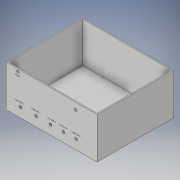
# Autodesk Inventor part: SeniorProjects
Saved by Autodesk Inventor 2019 (Build 230136000, 136)
## iProperties
Created: 2019-02-05
Part Number: SeniorProjects
Material: Generic
Document SubType Name: Modeling
Designer: Austin
Density: 1 g/cm^3
Appearance: Default
Author: Austin
Autodesk Inventor part; units mm, degrees
ref_plane "YZ Plane" through (0, 0, 0) normal (1, 0, 0) x (0, 1, 0)
ref_plane "XZ Plane" through (0, 0, 0) normal (0, 1, 0) x (-1, 0, 0)
ref_plane "XY Plane" through (0, 0, 0) normal (0, 0, 1) x (1, 0, 0)
sketch "Sketch1" plane through (0, 0, 0) normal (0, 1, 0) x (-1, 0, 0)
  line L0 (0, 0) -> (-203.2, 0)
  line L1 (-203.2, 0) -> (-203.2, 171.45)
  line L2 (-203.2, 171.45) -> (0, 171.45)
  line L3 (0, 171.45) -> (0, 0)
  dimension "d47" = 203.2
  dimension "d48" = 171.45
  constraints: 8 end point, 2 parallel, 1 horizontal, 1 perpendicular
  measures "d47" distance of L1.end L2.end
  measures "d48" distance of L0.end L1.end
extrude "Extrusion1" add sketch "Sketch1" along normal blind 2.54
sketch "Sketch2" plane through (0, 2.54, 0) normal (0, 1, 0) x (1, 0, 0)
  point P0 (0, 0)
sketch "Sketch3" plane through (203.2, 0, 171.45) normal (1, 0, 0) x (0, 0, -1)
  line L0 (171.45, 2.54) -> (0, 2.54) projected
  line L1 (0, 2.54) -> (171.4319, 2.54)
  line L2 (171.4319, 2.54) -> (171.4319, 92.0353)
  line L3 (171.4319, 92.0353) -> (0, 92.0353)
  line L4 (0, 92.0353) -> (0, 2.54)
  point P0 (171.45, 0)
  constraints: 8 end point, 2 parallel, 1 horizontal, 1 perpendicular
extrude "Extrusion2" add sketch "Sketch3" against normal blind 2.54
sketch "Sketch4" plane through (0, 0, 171.45) normal (0, 0, 1) x (1, 0, 0)
  line L0 (200.66, 2.54) -> (0, 2.54) projected
  line L1 (200.66, 92.0353) -> (200.66, 2.54) projected
  line L2 (0, 2.54) -> (200.66, 2.54)
  line L3 (200.66, 2.54) -> (200.66, 92.0353)
  line L4 (200.66, 92.0353) -> (0, 92.0353)
  line L5 (0, 92.0353) -> (0, 2.54)
  point P0 (0, 0)
  constraints: 8 end point, 2 parallel, 1 horizontal, 1 perpendicular
extrude "Extrusion3" add sketch "Sketch4" against normal blind 2.54
sketch "Sketch6" plane through (0, 0, 0) normal (-1, 0, 0) x (0, 0, 1)
  line L0 (168.91, 2.54) -> (168.91, 92.0353) projected
  line L1 (0, 2.54) -> (168.91, 2.54) projected
  line L2 (168.91, 92.0353) -> (0, 92.0353)
  line L3 (0, 92.0353) -> (0, 2.54)
  line L4 (0, 2.54) -> (168.91, 2.54)
  line L5 (168.91, 2.54) -> (168.91, 92.0353)
  point P0 (0, 0)
  constraints: 8 end point, 2 parallel, 1 horizontal, 1 perpendicular
extrude "Extrusion5" add sketch "Sketch6" against normal blind 2.54
sketch "Sketch7" plane through (203.2, 0, 0) normal (0, 0, -1) x (-1, 0, 0)
  line L0 (2.54, 2.54) -> (2.54, 92.0353) projected
  line L1 (200.66, 2.54) -> (2.54, 2.54) projected
  line L2 (2.54, 92.0353) -> (200.66, 92.0353)
  line L3 (200.66, 92.0353) -> (200.66, 2.54)
  line L4 (200.66, 2.54) -> (2.54, 2.54)
  line L5 (2.54, 2.54) -> (2.54, 92.0353)
  line L6 (0, 92.0353) -> (2.54, 92.0353) projected
  line L7 (2.54, 92.0353) -> (2.54, 2.54)
  line L8 (0, 2.54) -> (0, 92.0353)
  line L9 (0, 93.2997) -> (0, 2.54)
  point P0 (203.2, 0)
  constraints: 14 end point, 2 parallel, 2 vertical, 1 horizontal, 1 perpendicular
extrude "Extrusion6" add sketch "Sketch7" against normal blind 2.54
sketch "Sketch9" plane through (0, 0, 171.45) normal (0, 0, 1) x (1, 0, 0)
  point P0 (0, 0)
  point P1 (31.7946, 20.6466)
  point P2 (67.0265, 20.6942)
  point P3 (99.0634, 20.4536)
  point P4 (128.2662, 20.7894)
  point P5 (156.2119, 20.9564)
  point P6 (25.7932, 86.1813)
sketch "Sketch13" plane through (0, 0, 171.45) normal (0, 0, 1) x (1, 0, 0)
  line L0 (19.8638, 80.6749) -> (31.2777, 80.6749) construction
  line L1 (31.2777, 80.6749) -> (31.2777, 77.5627) construction
  line L2 (31.2777, 77.5627) -> (19.8638, 77.5627) construction
  line L3 (19.8638, 77.5627) -> (19.8638, 80.6749) construction
  line L4 (20.222, 32.0119) -> (39.4189, 32.0119) construction
  line L5 (39.4189, 32.0119) -> (39.4189, 26.7629) construction
  line L6 (39.4189, 26.7629) -> (20.222, 26.7629) construction
  line L7 (20.222, 26.7629) -> (20.222, 32.0119) construction
  line L8 (56.7268, 32.8288) -> (81.0219, 32.8288) construction
  line L9 (81.0219, 32.8288) -> (81.0219, 30.5168) construction
  line L10 (81.0219, 30.5168) -> (56.7268, 30.5168) construction
  line L11 (56.7268, 30.5168) -> (56.7268, 32.8288) construction
  line L12 (91.3347, 32.275) -> (110.5316, 32.275) construction
  line L13 (110.5316, 32.275) -> (110.5316, 27.6577) construction
  line L14 (110.5316, 27.6577) -> (91.3347, 27.6577) construction
  line L15 (91.3347, 27.6577) -> (91.3347, 32.275) construction
  line L16 (117.5581, 32.4429) -> (136.7551, 32.4429) construction
  line L17 (136.7551, 32.4429) -> (136.7551, 27.2492) construction
  line L18 (136.7551, 27.2492) -> (117.5581, 27.2492) construction
  line L19 (117.5581, 27.2492) -> (117.5581, 32.4429) construction
  line L20 (146.3399, 32.2758) -> (165.5369, 32.2758) construction
  line L21 (165.5369, 32.2758) -> (165.5369, 27.3704) construction
  line L22 (165.5369, 27.3704) -> (146.3399, 27.3704) construction
  line L23 (146.3399, 27.3704) -> (146.3399, 32.2758) construction
  point P0 (0, 0)
  constraints: 12 other
sketch "Sketch14" plane through (203.2, 0, 0) normal (0, 0, -1) x (-1, 0, 0)
  line L0 (14.8871, 35.1552) -> (31.5103, 35.1552) construction
  line L1 (31.5103, 35.1552) -> (31.5103, 32.043) construction
  line L2 (31.5103, 32.043) -> (14.8871, 32.043) construction
  line L3 (14.8871, 32.043) -> (14.8871, 35.1552) construction
  point P0 (203.2, 0)
  constraints: 2 other
sketch "Sketch15" plane through (203.2, 0, 0) normal (0, 0, -1) x (-1, 0, 0)
  line L0 (15.4634, 20.3313) -> (29.8713, 20.3313)
  line L1 (29.8713, 20.3313) -> (29.8713, 10.2457)
  line L2 (29.8713, 10.2457) -> (15.4634, 10.2457)
  line L3 (15.4634, 10.2457) -> (15.4634, 20.3313)
  line L4 (2.54, 2.54) -> (200.66, 2.54) projected
  point P0 (203.2, 0)
  dimension "d43" = 17.7913
  dimension "d44" = 7.7058
  constraints: 8 end point, 2 parallel, 1 horizontal, 1 perpendicular
  measures "d43" distance from line of L4 L0.start
  measures "d44" distance between parallel lines of L4 L2
extrude "Extrusion8" cut sketch "Sketch15" against normal blind 5.08
sketch "Sketch16" plane through (0, 0, 171.45) normal (0, 0, 1) x (1, 0, 0)
  point P0 (0, 0)
sketch "Sketch17" plane through (0, 0, 171.45) normal (0, 0, 1) x (1, 0, 0)
  point P0 (0, 0)
  point P1 (155.2724, 77.016)
hole "Hole4" at (155.2724, 77.016, 171.45) direction (0, 0, -1) diameter 6.35 depth 12.7 start extended yes
hole "Hole5" at (31.7946, 20.6466, 171.45) at (67.0265, 20.6942, 171.45) at (99.0634, 20.4536, 171.45) at (128.2662, 20.7894, 171.45) at (25.7932, 86.1813, 171.45) at (156.2119, 20.9564, 171.45) direction (0, 0, 1) diameter 6.35 end through all start extended yes
body "Solid1"
